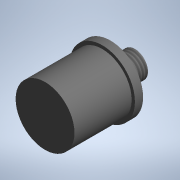
# Autodesk Inventor part: LZ80_Zapfen
Saved by Autodesk Inventor 2021.2 (Build 252289000, 289)
## iProperties
Part Number: LZ80_Zapfen
Material: Genérico
Catalog Web Link: www.cadenas.de
Description: LZ80 Zapfen-Bauteil LZ80
Vendor: ROSEKRIEGER
Document SubType Name: Modeling
Designer: partserver
Manufacturer: ROSEKRIEGER
Mass: 48.2228 g
Surface Area: 91.6484 cm^2
Volume: 48.2228 cm^3
Density: 1 g/cm^3
Appearance: PSOLRGB-128-128-128
Category: PARTsolutions
Company: ROSEKRIEGER
PSOL_IDENT_0: {$CADENAS_DATA\23d-libs\rose_krieger\linearkomponenten\pool_lineartechnik\_hubsaeule_zyliinder\elekt
PSOL_IDENT_1: rozylinder\elekzyl_lz80\lz80_zapfen.prj},167 {VTYP=3D},{NB=LZ80_Zapfen},{LINA=LZ80_Zapfen},{NN=LZ80
PSOL_IDENT_2: Zapfen},{DATE=02.12.2020 11:16:41},{GEOMDATE=22.06.2012 05:25:00},{VERSION=},{LINEID=10},{WBVAR=},{W
PSOL_IDENT_3: BNUMERIC=}  {NB=LZ80_Zapfen},{LINA=LZ80_Zapfen},{KT=DUMMY},{IDNR=},{ARTIKEL=LZ80_Zapfen},{ZAPFENLAEN=
PSOL_IDENT_4: 35.000},{ZAPFENDURC=16.000},{ZENDURCH=36.000},{ZENLAENG=15.000},{BUNDDURCH=40.000},{BUNDHOE=5.000},{
PSOL_IDENT_5: FASE=1.200},{GWNS=16.000},{GWKS=13.546},{SW=8.000},{TSS=12.400}
NB: LZ80_Zapfen
NN: LZ80 Zapfen
NT: Bauteil LZ80
NBSYN: $ARTIKEL.
LINA: LZ80_Zapfen
CATALOG: RK Rose+Krieger
ARTIKEL: LZ80_Zapfen
ZAPFENLAEN: 35
ZAPFENDURC: 16
ZENDURCH: 36
ZENLAENG: 15
BUNDDURCH: 40
BUNDHOE: 5
FASE: 1.2
GWNS: 16
GWKS: 13.546
SW: 8
TSS: 12.4
SUPPLIER: ROSEKRIEGER
ARTICLENO: LZ80_Zapfen
BOMINFO: LZ80_Zapfen
CREATOR: CADENAS GmbH
Title: LZ80_Zapfen
Author: Cadenas PARTsolutions
Comments: Bauteil LZ80
Autodesk Inventor part; units mm, degrees
ref_plane "YZ Plane" through (0, 0, 0) normal (1, 0, 0) x (0, 1, 0)
ref_plane "XZ Plane" through (0, 0, 0) normal (0, 1, 0) x (-1, 0, 0)
ref_plane "XY Plane" through (0, 0, 0) normal (0, 0, 1) x (1, 0, 0)
sketch "Skizze_1" plane through (0, 0, 0) normal (0, 0, 1) x (1, 0, 0)
  line L0 (0, -35) -> (0, 40)
  line L1 (0, 40) -> (6.773, 40)
  line L2 (6.773, 40) -> (8, 38.773)
  line L3 (8, 38.773) -> (8, 5)
  line L4 (8, 5) -> (20, 5)
  line L5 (20, 5) -> (20, 0)
  line L6 (20, 0) -> (18, 0)
  line L7 (18, 0) -> (18, -35)
  line L8 (18, -35) -> (0, -35)
  line L9 (0, -35) -> (0, 40)
  constraints: 20 end point
revolve "Revolution1" add sketch "Skizze_1" angle 360 about axis through (0, -35, 0) along (0, -1, 0)
thread "Thread1" size "M16x2" class "6g" standard "ISO Metric profile" full length
sketch "Skizze_2" plane through (0, 40, 0) normal (0, 1, 0) x (1, 0, 0)
  line L0 (-4, -2.3094) -> (0, -4.6188)
  line L1 (0, -4.6188) -> (4, -2.3094)
  line L2 (4, -2.3094) -> (4, 2.3094)
  line L3 (4, 2.3094) -> (0, 4.6188)
  line L4 (0, 4.6188) -> (-4, 2.3094)
  line L5 (-4, 2.3094) -> (-4, -2.3094)
  constraints: 12 end point
extrude "Extrusion1" cut sketch "Skizze_2" against normal blind 12.4
ref_plane "EPHUB_XY" through (0, 5, 0) normal (0, 1, 0) x (1, 0, 0)
ref_plane "EPHUB_YZ" through (0, 5, 0) normal (1, 0, 0) x (0, 0, -1)
ref_plane "EPHUB_ZX" through (0, 5, 0) normal (0, 0, -1) x (0, 1, 0)
ref_plane "EPZAPFEN_XY" through (0, 0, 0) normal (0, 1, 0) x (1, 0, 0)
ref_plane "EPZAPFEN_YZ" through (0, 0, 0) normal (1, 0, 0) x (0, 0, -1)
ref_plane "EPZAPFEN_ZX" through (0, 0, 0) normal (0, 0, -1) x (0, 1, 0)
sketch "Boceto3" plane through (0, 5, 0) normal (0, 1, 0) x (1, 0, 0)
  point P0 (0, 0)
sketch "Boceto4" plane through (0, 40, 0) normal (0, 1, 0) x (1, 0, 0)
  circle A0 centre (0, 0) radius 8
  dimension "d7" = 16
  constraints: 1 centre point, 1 coincident
  measures "d7" diameter of A0
extrude "Extrusión2" cut sketch "Boceto4" against normal blind 20
body "Solid1"
